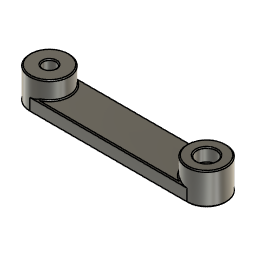
Rotary Link v2 (Autodesk Fusion 360 design; units mm, degrees)
Autodesk Fusion 360 part; units mm, degrees
sketch "Sketch1" plane through (0, 0, 0) normal (0, 0, 1) x (1, 0, 0)
  circle A0 centre (0, 0) radius 3.275
  circle A1 centre (0, 0) radius 10
  circle A2 centre (80, 0) radius 3.275
  circle A3 centre (80, 0) radius 10
  line L0 (0, 10) -> (80, 10)
  line L1 (0, -10) -> (80, -10)
  dimension "d2" = 6.55
  dimension "d3" = 20
  dimension "d5" = 6.55
  dimension "d6" = 20
  dimension "d7" = 80
  constraint coincident A0.centre A1.centre
  constraint concentric A0 A1
  constraint concentric A2 A3
  constraint coincident A1 L0.start
  constraint coincident A3 L0.end
  constraint tangent A3 L0
  constraint coincident A1 L1.start
  constraint coincident A3 L1.end
  constraint tangent A3 L1
  constraint tangent A1 L1
  constraint tangent A1 L0
  constraint horizontal A0.centre A2.centre
  measures "d2" diameter of A0
  measures "d3" diameter of A1
  measures "d5" diameter of A2
  measures "d6" diameter of A3
  measures "d7" horizontal distance of A0.centre A2.centre
extrude "Extrude1" add sketch "Sketch1" along normal blind 7 contours A1 A3 L0 L1
extrude "Extrude2" add sketch "Sketch1" along normal blind 16 contours A1 | A3
sketch "Sketch4" plane through (0, 0, 16) normal (0, 0, 1) x (-1, 0, 0)
  circle A0 centre (0, 0) radius 3.275
  circle A1 centre (0, 0) radius 10
  line L0 (-3.3198, 5.75) -> (-6.6395, 0)
  line L1 (-6.6395, 0) -> (-3.3198, -5.75)
  line L2 (-3.3198, -5.75) -> (3.3198, -5.75)
  line L3 (3.3198, -5.75) -> (6.6395, 0)
  line L4 (6.6395, 0) -> (3.3198, 5.75)
  line L5 (3.3198, 5.75) -> (-3.3198, 5.75)
  dimension "d26" = 5.75
  constraint coincident A0.centre A1.centre
  constraint horizontal L5
  measures "d26" distance of A0.centre L5
extrude "Extrude5" [suppressed]
sketch "Sketch3" plane through (0, 0, 16) normal (0, 0, 1) x (-1, 0, 0)
  line L0 (-3.3198, 5.75) -> (-6.6395, 0)
  line L1 (-6.6395, 0) -> (-3.3198, -5.75)
  line L2 (-3.3198, -5.75) -> (3.3198, -5.75)
  line L3 (3.3198, -5.75) -> (6.6395, 0)
  line L4 (6.6395, 0) -> (3.3198, 5.75)
  line L5 (3.3198, 5.75) -> (-3.3198, 5.75)
  circle A0 centre (-80, 0) radius 10
  circle A1 centre (0, 0) radius 10
  circle A2 centre (-80, 0) radius 3.275
  circle A3 centre (0, 0) radius 3.275
  dimension "d23" = 5.75
  measures "d23" distance of A1.centre L5
chamfer "Chamfer5" distance 0.5 angle 45 4 faces at (7.7089, 0.6595, 16) (87.7089, 0.6595, 16) (50.0186, 0, 7) (27.6502, 7.1403, 0)
chamfer "Chamfer6" [suppressed]
sketch "Sketch5" plane through (0, 0, 16) normal (0, 0, 1) x (-1, 0, 0)
  circle A0 centre (-80, 0) radius 3.775
  circle A1 centre (-80, 0) radius 9.5
  circle A2 centre (-80, 0) radius 5
  dimension "d31" = 10
  constraint concentric A0 A2
  measures "d31" diameter of A2
extrude "Extrude6" cut sketch "Sketch5" against normal blind 6.5 contours A0 | A2
chamfer "Chamfer7" distance 0.5 angle 45 2 edges at (84.6616, -1.8081, 16) (76.9466, -1.1843, 9.5)
equation "ScrewHoleSize = 6.4 mm"
equation "d3 = OuterDiameter"
equation "LinkLength = 80 mm"
equation "d6 = OuterDiameter"
equation "d7 = LinkLength"
equation "d8 = LinkThickness"
equation "d10 = PivotExtrudeDepth"
equation "OuterDiameter = 20 mm"
equation "PivotExtrudeDepth = 16 mm"
equation "LinkThickness = 7 mm"
equation "d23 = ( 11.5 / 2 ) * 1 mm"
equation "d26 = ( 11.5 / 2 ) * 1 mm"
